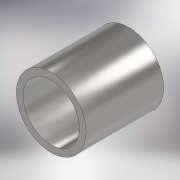
# Autodesk Inventor part: Sleeve_
Saved by Autodesk Inventor 2020 (Build 240168000, 168)
## iProperties
Created: 2019-05-19
Part Number: Sleeve_
Material: Steel, Mild
Document SubType Name: Modeling
Designer: chitl
Density: 7.85 g/cm^3
Appearance: Semi-Polished
Author: chitl
Autodesk Inventor part; units mm, degrees
ref_plane "YZ Plane" through (0, 0, 0) normal (1, 0, 0) x (0, 1, 0)
ref_plane "XZ Plane" through (0, 0, 0) normal (0, 1, 0) x (-1, 0, 0)
ref_plane "XY Plane" through (0, 0, 0) normal (0, 0, 1) x (1, 0, 0)
sketch "Sketch1" plane through (0, 0, 0) normal (0, 0, 1) x (1, 0, 0)
  circle A0 centre (0, 0) radius 6.9088
  circle A1 centre (0, 0) radius 8.5598
  dimension "d0" = 13.8176
  dimension "d1" = 1.651
  constraints: 2 centre point, 1 coincident
  measures "d0" diameter of A0
  measures "d1" radial gap between concentric circles of A0 A1
extrude "Extrusion1" add sketch "Sketch1" along normal blind 19.05
body "Solid1"
